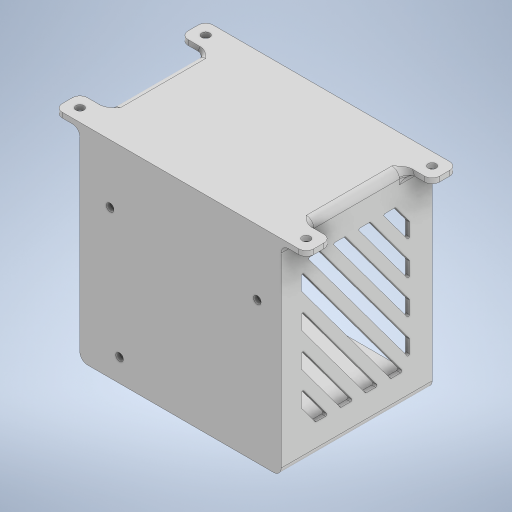
# Autodesk Inventor part: Caja2
Saved by Autodesk Inventor 2024 (Build 280153000, 153)
## iProperties
Created: 2023-04-03
Part Number: Caja2
Material: Genérico
Document SubType Name: Modeling
Designer: sergi
Density: 1 g/cm^3
Appearance: Valor por defecto
Author: sergi
Autodesk Inventor part; units mm, degrees
ref_plane "YZ Plane" through (0, 0, 0) normal (1, 0, 0) x (0, 1, 0)
ref_plane "XZ Plane" through (0, 0, 0) normal (0, 1, 0) x (-1, 0, 0)
ref_plane "XY Plane" through (0, 0, 0) normal (0, 0, 1) x (1, 0, 0)
sketch "Boceto1" plane through (0, 0, 0) normal (0, 0, 1) x (1, 0, 0)
  circle A0 centre (-35.8, -35.8) radius 2.125 projected
  circle A1 centre (35.8, 35.8) radius 2.125 projected
  circle A2 centre (35.8, -35.8) radius 2.125 projected
  circle A3 centre (-35.8, 35.8) radius 2.125 projected
  line L0 (-40, -40) -> (-40, 40) projected
  line L1 (40, -40) -> (-40, -40) projected
  line L2 (40, 40) -> (40, -40) projected
  line L3 (-40, 40) -> (40, 40) projected
  line L4 (-40, 40) -> (40, 40)
  line L5 (40, 40) -> (40, -40)
  line L6 (40, -40) -> (-40, -40)
  line L7 (-40, -40) -> (-40, 40)
  line L8 (-41, -41) -> (-41, 41)
  line L9 (-41, 41) -> (41, 41)
  line L10 (41, 41) -> (41, -41)
  line L11 (41, -41) -> (-41, -41)
  point P0 (0, 0)
  dimension "d22" = 1
  constraints: 16 end point, 2 parallel, 1 horizontal, 1 perpendicular, 3 other
  measures "d22" distance between parallel lines of L1 L11
extrude "Extrusión1" add sketch "Boceto1" along normal blind 60 contours A0 | A1 | A2 | A3 | L0 L3 L2 L1
sketch "Boceto2" plane through (0, 0, 0) normal (0, 0, -1) x (-1, 0, 0)
  circle A0 centre (35.8, 35.8) radius 2.125 projected
  circle A1 centre (35.8, -35.8) radius 2.125 projected
  circle A2 centre (-35.8, -35.8) radius 2.125 projected
  circle A3 centre (-35.8, 35.8) radius 2.125 projected
  point P0 (0, 0)
hole "Agujero1" at (-35.8, 35.8, 0) at (-35.8, -35.8, 0) at (35.8, -35.8, 0) at (35.8, 35.8, 0) direction (0, 0, 1) diameter 4.25 depth 10
shell "Vaciado1" thickness 1.6 removed faces 2 at (11.4636, -11.4031, 0) at (13.3333, 40, 20)
sketch "Boceto3" plane through (37.8, 37.8, 58.4) normal (0, 0, -1) x (-1, 0, 0)
  circle A0 centre (65.77, -19.059) radius 1.4999 projected
  circle A1 centre (62.025, -68.7162) radius 1.5 projected
  line L0 (76.2, 2.2) -> (76.2, -76.2) projected
  line L1 (-0.6, -76.2) -> (-0.6, 2.2) projected
  line L2 (76.2, -76.2) -> (-0.6, -76.2) projected
  circle A2 centre (7.8236, -54.3604) radius 1.5 projected
  circle A3 centre (7.2748, -21.6806) radius 1.5001 projected
  circle A4 centre (65.77, -19.059) radius 3
  circle A5 centre (62.025, -68.7162) radius 3
  circle A6 centre (7.8236, -54.3604) radius 3
  circle A7 centre (7.2748, -21.6806) radius 3
  line L3 (-0.6, 2.2) -> (76.2, 2.2) projected
  point P0 (37.8, -37.8)
  dimension "d10" = 6
  dimension "d11" = 6
  dimension "d12" = 6
  dimension "d13" = 6
  constraints: 4 centre point, 4 coincident
  measures "d10" diameter of A4
  measures "d11" diameter of A5
  measures "d12" diameter of A6
  measures "d13" diameter of A7
extrude "Extrusión2" add sketch "Boceto3" along normal blind 5 contours A4 | A5 | A6 | A7
fillet "Empalme1" radius 2 4 edges at (-21.225, -30.9162, 58.4) (32.9764, -16.5604, 58.4) (33.5252, 16.1194, 58.4) (-24.97, 18.741, 58.4)
sketch "Boceto4" plane through (-38.4, -38.4, 58.4) normal (1, 0, 0) x (0, 0, -1)
  line L0 (14.2955, 15.5019) -> (14.2955, 22.9876) projected
  line L1 (14.2955, 22.9876) -> (7, 23.1181) projected
  line L2 (7, 15.5019) -> (14.2955, 15.5019) projected
  line L3 (14.2955, 15.5019) -> (7, 15.5019)
  line L4 (7, 15.5019) -> (7, 23.1181)
  line L5 (7, 23.1181) -> (14.2955, 23.1181)
  line L6 (14.2955, 23.1181) -> (14.2955, 15.5019)
  line L7 (6, 24.1181) -> (6, 14.5019)
  line L8 (6, 14.5019) -> (15.2955, 14.5019)
  line L9 (15.2955, 14.5019) -> (15.2955, 24.1181)
  line L10 (15.2955, 24.1181) -> (6, 24.1181)
  point P0 (58.4, 38.4)
  point P1 (14.2955, 22.9876)
  point P2 (10.9796, 28.9019)
  dimension "d17" = 1
  constraints: 16 end point, 4 parallel, 2 perpendicular, 1 horizontal, 3 other
  measures "d17" distance between parallel lines of L4 L7
extrude "Extrusión3" cut sketch "Boceto4" against normal blind 5 contours L2 L4 L1 L0 | L1 L5 L6 | L10 L9 L8 L7
sketch "Boceto5" plane through (-40, 40, 0) normal (0, 1, 0) x (1, 0, 0)
  line L0 (0, -60) -> (80, -60) projected
  line L1 (0, -60) -> (80, -60)
  line L2 (80, -60) -> (80, 15.124)
  line L3 (80, 15.124) -> (0, 15.124)
  line L4 (0, 15.124) -> (0, -60)
  point P0 (40, 0)
  constraints: 8 end point, 2 parallel, 1 horizontal, 1 perpendicular
extrude "Extrusión4" add sketch "Boceto5" along normal blind 2
sketch "Boceto6" plane through (-40, 42, 0) normal (0, 1, 0) x (1, 0, 0)
  line L0 (80, 15.124) -> (0, 15.124) projected
  line L1 (80, -60) -> (80, 15.124) projected
  line L2 (0, 15.124) -> (80, 15.124)
  line L3 (80, 15.124) -> (80, 12.124)
  line L4 (80, 12.124) -> (0, 12.124)
  line L5 (0, 12.124) -> (0, 15.124)
  point P0 (40, 0)
  dimension "d25" = 3
  constraints: 8 end point, 2 parallel, 1 horizontal, 1 perpendicular, 1 point on line
  measures "d25" distance of L2.end L3.end
extrude "Extrusión5" add sketch "Boceto6" along normal blind 15
sketch "Boceto7" plane through (40, 40, -15.124) normal (0, 0, -1) x (-1, 0, 0)
  line L0 (0, 2) -> (80, 2) projected
  line L1 (80, 0) -> (80, 17) projected
  point P0 (40, -40)
  point P1 (70, 11.3)
  dimension "d28" = 9.3
  dimension "d29" = 10
  measures "d28" distance from line of L0 point (70, 11.3)
  measures "d29" distance from line of L1 point (70, 11.3)
hole "Agujero2" at (-30, 51.3, -15.124) direction (0, 0, 1) diameter 5 depth 10
sketch "Boceto8" plane through (40, 40, -15.124) normal (0, 0, -1) x (-1, 0, 0)
  line L0 (0, 2) -> (80, 2) projected
  line L1 (0, 0) -> (0, 17) projected
  point P0 (40, -40)
  point P1 (10, 11.3)
  dimension "d37" = 9.3
  dimension "d38" = 10
  measures "d37" distance from line of L0 point (10, 11.3)
  measures "d38" distance from line of L1 point (10, 11.3)
hole "Agujero3" at (30, 51.3, -15.124) direction (0, 0, 1) diameter 5 depth 10
fillet "Empalme2" radius 3 6 edges at (-40, 42, 23.938) (-40, -40, 30) (40, 42, 23.938) (40, -40, 30) (-40, 57, -13.624) (40, 57, -13.624)
sketch "Boceto9" plane through (-38.4, -33.1325, 0) normal (1, 0, 0) x (0, 0, -1)
  line L0 (-32.0511, 38.9222) -> (-32.0511, 48.6464) projected
  line L1 (-32.0511, 48.6464) -> (-43.4, 48.6464) projected
  line L2 (-58.4, 73.1325) -> (0, 73.1325) projected
  line L3 (-32.0511, 48.6464) -> (-7.565, 48.6464) construction
  line L4 (-42.05, 61.453) -> (-53.55, 61.453)
  line L5 (-53.55, 61.453) -> (-53.55, 70.953)
  line L6 (-53.55, 70.953) -> (-42.05, 70.953)
  line L7 (-42.05, 70.953) -> (-42.05, 61.453)
  line L8 (-58.4, 73.1325) -> (-58.4, -5.2675) projected
  point P0 (0, 33.1325)
  point P1 (-53.55, 66.203)
  dimension "d50" = 11.5
  dimension "d145" = 4.85
  dimension "d146" = 9.5
  constraints: 10 end point, 2 horizontal, 2 parallel, 1 midpoint, 1 perpendicular
  measures "d50" distance of L5.end L6.end
  measures "d145" distance between parallel lines of L8 L5
  measures "d146" distance of L6.end L4.start
extrude "Extrusión6" cut sketch "Boceto9" against normal blind 15
fillet "Empalme4" radius 2 6 edges at (33.1325, -38.4, 5.8) (38.4, -33.1325, 5.8) (38.4, 33.1325, 5.8) (-38.4, 33.1325, 5.8) (-33.1325, -38.4, 5.8) (-38.4, -33.1325, 5.8)
sketch "Boceto11" plane through (-38.4, -38.4, 58.4) normal (0, 1, 0) x (1, 0, 0)
  line L0 (17.175, 5) -> (11.175, 5) projected
  line L1 (17.175, 5) -> (67.175, 5)
  line L2 (67.175, 5) -> (67.175, 13)
  line L3 (67.175, 13) -> (17.175, 13)
  line L4 (17.175, 13) -> (17.175, 5)
  line L5 (71.3764, 5) -> (65.3764, 5) projected
  point P0 (38.4, 58.4)
  dimension "d58" = 50
  dimension "d59" = 8
  constraints: 8 end point, 2 parallel, 1 horizontal, 1 perpendicular
  measures "d58" distance of L3.end L2.end
  measures "d59" distance of L2.end L1.end
extrude "Extrusión8" cut sketch "Boceto11" against normal blind 4.5
ref_plane "Plano de trabajo1" through (0, 0, 0) normal (0, 0, -1) x (-1, 0, 0)
split "Dividir1" plane through (0, 0, 0) removes the side toward (0, 0, -1)
sketch "Boceto12" plane through (40, -37, 0) normal (1, 0, 0) x (0, 0, -1)
  line L0 (0, 0) -> (-60, 0) projected
  line L1 (0, 0) -> (0, 76) projected
  line L2 (-60, 76) -> (0, 76) projected
  line L3 (-60, 0) -> (-60, 76) projected
  line L4 (0, 106.0697) -> (0, -25.6754) projected
  line L5 (-51.3248, 9) -> (-9, 9)
  line L6 (-9, 9) -> (-9, 67)
  line L7 (-9, 67) -> (-50, 67)
  line L8 (-52, 0) -> (-52, 76)
  line L9 (-9, 9) -> (-52, 67)
  line L10 (-11.4897, 9) -> (-53.6066, 65.8089)
  line L11 (-9, 12.3582) -> (-50.3934, 68.1911)
  line L12 (-7.438, 16.9677) -> (-47.1801, 70.5734)
  line L13 (-4.2248, 19.3499) -> (-43.9669, 72.9556)
  line L14 (-1.0115, 21.7322) -> (-40.7536, 75.3378)
  line L15 (2.2017, 24.1144) -> (-37.5404, 77.7201)
  line L16 (5.415, 26.4967) -> (-34.3271, 80.1023)
  line L17 (8.6282, 28.8789) -> (-31.1139, 82.4845)
  line L18 (-16.4691, 9) -> (-56.8199, 63.4266)
  line L19 (-20.291, 7.4388) -> (-60.0331, 61.0444)
  line L20 (-23.5043, 5.0565) -> (-63.2464, 58.6622)
  line L21 (-26.7175, 2.6743) -> (-66.4596, 56.2799)
  line L22 (-29.9307, 0.2921) -> (-69.6729, 53.8977)
  line L23 (-33.144, -2.0902) -> (-72.8861, 51.5155)
  line L24 (-36.3572, -4.4724) -> (-76.0994, 49.1332)
  line L25 (11.8415, 31.2611) -> (-27.9006, 84.8668)
  line L26 (15.0547, 33.6434) -> (-24.6874, 87.249)
  line L27 (-39.5705, -6.8546) -> (-79.3126, 46.751)
  point P0 (-42, 9)
  point P1 (-41.366, 9)
  point P2 (-52, 23.3435)
  point P3 (-9, 19.0746)
  point P4 (-44.5309, 67)
  point P5 (-49.5103, 67)
  point P6 (-9, 13.0443)
  point P7 (-9, 32.5073)
  point P8 (-34.5721, 67)
  point P9 (-39.5515, 67)
  point P10 (-9, 25.791)
  point P11 (-9, 45.9401)
  point P12 (-24.6134, 67)
  point P13 (-29.5928, 67)
  point P14 (-9, 39.2237)
  point P15 (-19.634, 67)
  point P16 (-9, 52.6565)
  point P17 (-52, 56.9254)
  point P18 (-15.9032, 9)
  point P19 (-11.3011, 9)
  point P20 (-52, 63.6418)
  point P21 (-52, 43.4927)
  point P22 (-26.4279, 9)
  point P23 (-21.4485, 9)
  point P24 (-52, 50.209)
  point P25 (-52, 30.0599)
  point P26 (-36.3866, 9)
  point P27 (-31.4072, 9)
  point P28 (-52, 36.7763)
  point P29 (-52, 16.6271)
  point P30 (-46.3454, 9)
  point P31 (-9, 59.3729)
  point P32 (-14.6546, 67)
  dimension "d83" = 9
  dimension "d84" = 8
  dimension "L" = 2
  dimension "d86" = 2
  dimension "d87" = 4
  dimension "d88" = 4
  dimension "d89" = 4
  dimension "d90" = 4
  dimension "d91" = 4
  dimension "d92" = 4
  dimension "d93" = 4
  dimension "d94" = 4
  dimension "d95" = 4
  dimension "d96" = 4
  dimension "d97" = 4
  dimension "d98" = 4
  dimension "d99" = 4
  dimension "d140" = 4
  dimension "d141" = 4
  dimension "d142" = 4
  constraints: 46 end point, 19 parallel, 6 point on line, 1 other
  measures "d83" distance between parallel lines of L0 L5
  measures "d84" distance between parallel lines of L3 L8
  measures "L" distance between parallel lines of L9 L10
  measures "d86" distance between parallel lines of L9 L11
  measures "d87" distance between parallel lines of L11 L12
  measures "d88" distance between parallel lines of L12 L13
  measures "d89" distance between parallel lines of L13 L14
  measures "d90" distance between parallel lines of L14 L15
  measures "d91" distance between parallel lines of L15 L16
  measures "d92" distance between parallel lines of L16 L17
  measures "d93" distance between parallel lines of L10 L18
  measures "d94" distance between parallel lines of L18 L19
  measures "d95" distance between parallel lines of L19 L20
  measures "d96" distance between parallel lines of L20 L21
  measures "d97" distance between parallel lines of L21 L22
  measures "d98" distance between parallel lines of L22 L23
  measures "d99" distance between parallel lines of L23 L24
  measures "d140" distance between parallel lines of L17 L25
  measures "d141" distance between parallel lines of L25 L26
  measures "d142" distance between parallel lines of L24 L27
extrude "Extrusión9" cut sketch "Boceto12" against normal up to surface (1.6 mm away) contours L8 L23 L5 L24 | L8 L21 L5 L22 | L15 L7 L16 L6 | L8 L19 L5 L20 | L6 L13 L7 L14 | L17 L7 L25 L6 | L8 L10 L5 L18 | L6 L11 L7 L12
fillet "Empalme5" radius 0.5 32 edges at (39.2, -17.9254, 9) (39.2, -28, 21.4485) (39.2, -28, 26.4279) (39.2, -28, 31.4072) (39.2, -28, 36.3866) (39.2, -28, 41.366) (39.2, -13.6565, 52) (39.2, -6.9401, 52) (39.2, -0.2237, 52) (39.2, 6.4927, 52) (39.2, 13.209, 52) (39.2, 19.9254, 52) (39.2, 26.6418, 52) (39.2, 30, 49.5103) (39.2, 30, 44.5309) (39.2, 30, 39.5515) (39.2, 30, 34.5721) (39.2, 30, 29.5928) (39.2, 30, 24.6134) (39.2, 30, 19.634) (39.2, 15.6565, 9) (39.2, 8.9401, 9) (39.2, 2.2237, 9) (39.2, -4.4927, 9) (39.2, -11.209, 9) (39.2, -24.6418, 9) (39.2, -28, 11.4897) (39.2, -28, 16.4691) (39.2, -28, 46.3454) (39.2, -20.3729, 52) (39.2, 30, 14.6546) (39.2, 22.3729, 9)
sketch "Boceto13" plane through (-40, -37, 0) normal (-1, 0, 0) x (0, 0, 1)
  line L0 (36.5365, 9.2022) -> (51.9017, 29.9272) construction
  arc A0 (51.9017, 29.9272) -> (52, 30.225) centre (51.5, 30.225) ccw construction
  line L1 (52, 30.225) -> (52, 35.2623) construction
  arc A1 (52, 35.2623) -> (51.0983, 35.5601) centre (51.5, 35.2623) ccw construction
  line L2 (51.0983, 35.5601) -> (31.9987, 9.7978) construction
  arc A2 (31.9987, 9.7978) -> (32.4004, 9) centre (32.4004, 9.5) ccw construction
  line L3 (32.4004, 9) -> (36.1349, 9) construction
  arc A3 (36.1349, 9) -> (36.5365, 9.2022) centre (36.1349, 9.5) ccw construction
  line L4 (28.5996, 67) -> (24.8651, 67) construction
  line L5 (9, 45.775) -> (9, 40.7377) construction
  line L6 (26.5778, 9.2022) -> (51.9017, 43.36) construction
  arc A4 (51.9017, 43.36) -> (52, 43.6578) centre (51.5, 43.6578) ccw construction
  line L7 (52, 43.6578) -> (52, 48.6951) construction
  arc A5 (52, 48.6951) -> (51.0983, 48.9929) centre (51.5, 48.6951) ccw construction
  line L8 (51.0983, 48.9929) -> (22.0399, 9.7978) construction
  arc A6 (22.0399, 9.7978) -> (22.4416, 9) centre (22.4416, 9.5) ccw construction
  line L9 (22.4416, 9) -> (26.1761, 9) construction
  arc A7 (26.1761, 9) -> (26.5778, 9.2022) centre (26.1761, 9.5) ccw construction
  line L10 (44.381, 66.7978) -> (9.0983, 19.2072) construction
  arc A8 (9.0983, 19.2072) -> (9, 18.9094) centre (9.5, 18.9094) ccw construction
  arc A9 (44.7827, 67) -> (44.381, 66.7978) centre (44.7827, 66.5) ccw construction
  line L11 (0, 0) -> (60, 0) construction
  line L12 (0, 0) -> (0, 76) construction
  line L13 (60, 76) -> (0, 76) construction
  line L14 (60, 0) -> (60, 76) construction
  line L15 (24.4635, 66.7978) -> (9.0983, 46.0728) construction
  arc A10 (9.0983, 46.0728) -> (9, 45.775) centre (9.5, 45.775) ccw construction
  arc A11 (9, 40.7377) -> (9.9017, 40.4399) centre (9.5, 40.7377) ccw construction
  line L16 (9.9017, 40.4399) -> (29.0013, 66.2022) construction
  arc A12 (29.0013, 66.2022) -> (28.5996, 67) centre (28.5996, 66.5) ccw construction
  arc A13 (24.8651, 67) -> (24.4635, 66.7978) centre (24.8651, 66.5) ccw construction
  line L17 (48.5172, 67) -> (44.7827, 67) construction
  line L18 (9, 59.2077) -> (9, 54.1705) construction
  line L19 (9.9017, 13.5744) -> (48.9188, 66.2022) construction
  arc A14 (48.9188, 66.2022) -> (48.5172, 67) centre (48.5172, 66.5) ccw construction
  line L20 (14.5047, 66.7978) -> (9.0983, 59.5055) construction
  arc A15 (9.0983, 59.5055) -> (9, 59.2077) centre (9.5, 59.2077) ccw construction
  arc A16 (9, 54.1705) -> (9.9017, 53.8727) centre (9.5, 54.1705) ccw construction
  line L21 (9.9017, 53.8727) -> (19.0425, 66.2022) construction
  arc A17 (19.0425, 66.2022) -> (18.6409, 67) centre (18.6409, 66.5) ccw construction
  line L22 (18.6409, 67) -> (14.9063, 67) construction
  arc A18 (14.9063, 67) -> (14.5047, 66.7978) centre (14.9063, 66.5) ccw construction
  line L23 (38.5584, 67) -> (34.8239, 67) construction
  arc A19 (34.8239, 67) -> (34.4222, 66.7978) centre (34.8239, 66.5) ccw construction
  line L24 (34.4222, 66.7978) -> (9.0983, 32.64) construction
  arc A20 (9.0983, 32.64) -> (9, 32.3422) centre (9.5, 32.3422) ccw construction
  line L25 (9, 32.3422) -> (9, 27.3049) construction
  arc A21 (9, 27.3049) -> (9.9017, 27.0071) centre (9.5, 27.3049) ccw construction
  line L26 (9.9017, 27.0071) -> (38.9601, 66.2022) construction
  arc A22 (38.9601, 66.2022) -> (38.5584, 67) centre (38.5584, 66.5) ccw construction
  line L27 (9, 18.9094) -> (9, 13.8722) construction
  arc A23 (9, 13.8722) -> (9.9017, 13.5744) centre (9.5, 13.8722) ccw construction
  line L28 (12.4828, 9) -> (16.2173, 9) projected
  arc A24 (16.2173, 9) -> (16.619, 9.2022) centre (16.2173, 9.5) ccw projected
  line L29 (16.619, 9.2022) -> (51.9017, 56.7928) projected
  arc A25 (51.9017, 56.7928) -> (52, 57.0906) centre (51.5, 57.0906) ccw projected
  line L30 (52, 57.0906) -> (52, 62.1278) projected
  arc A26 (52, 62.1278) -> (51.0983, 62.4256) centre (51.5, 62.1278) ccw projected
  line L31 (51.0983, 62.4256) -> (12.0812, 9.7978) projected
  arc A27 (12.0812, 9.7978) -> (12.4828, 9) centre (12.4828, 9.5) ccw projected
  line L32 (14.5047, 66.7978) -> (9.0983, 59.5055) projected
  arc A28 (9.0983, 59.5055) -> (9, 59.2077) centre (9.5, 59.2077) ccw projected
  line L33 (9, 59.2077) -> (9, 54.1705) projected
  arc A29 (9, 54.1705) -> (9.9017, 53.8727) centre (9.5, 54.1705) ccw projected
  line L34 (9.9017, 53.8727) -> (19.0425, 66.2022) projected
  arc A30 (19.0425, 66.2022) -> (18.6409, 67) centre (18.6409, 66.5) ccw projected
  line L35 (18.6409, 67) -> (14.9063, 67) projected
  arc A31 (14.9063, 67) -> (14.5047, 66.7978) centre (14.9063, 66.5) ccw projected
  line L36 (38.5584, 67) -> (34.8239, 67) projected
  arc A32 (34.8239, 67) -> (34.4222, 66.7978) centre (34.8239, 66.5) ccw projected
  line L37 (34.4222, 66.7978) -> (9.0983, 32.64) projected
  arc A33 (9.0983, 32.64) -> (9, 32.3422) centre (9.5, 32.3422) ccw projected
  line L38 (9, 32.3422) -> (9, 27.3049) projected
  arc A34 (9, 27.3049) -> (9.9017, 27.0071) centre (9.5, 27.3049) ccw projected
  line L39 (9.9017, 27.0071) -> (38.9601, 66.2022) projected
  arc A35 (38.9601, 66.2022) -> (38.5584, 67) centre (38.5584, 66.5) ccw projected
  line L40 (26.5778, 9.2022) -> (51.9017, 43.36) projected
  arc A36 (51.9017, 43.36) -> (52, 43.6578) centre (51.5, 43.6578) ccw projected
  line L41 (52, 43.6578) -> (52, 48.6951) projected
  arc A37 (52, 48.6951) -> (51.0983, 48.9929) centre (51.5, 48.6951) ccw projected
  line L42 (51.0983, 48.9929) -> (22.0399, 9.7978) projected
  arc A38 (22.0399, 9.7978) -> (22.4416, 9) centre (22.4416, 9.5) ccw projected
  line L43 (22.4416, 9) -> (26.1761, 9) projected
  arc A39 (26.1761, 9) -> (26.5778, 9.2022) centre (26.1761, 9.5) ccw projected
  line L44 (48.5172, 67) -> (44.7827, 67) projected
  arc A40 (44.7827, 67) -> (44.381, 66.7978) centre (44.7827, 66.5) ccw projected
  line L45 (44.381, 66.7978) -> (9.0983, 19.2072) projected
  arc A41 (9.0983, 19.2072) -> (9, 18.9094) centre (9.5, 18.9094) ccw projected
  line L46 (9, 18.9094) -> (9, 13.8722) projected
  arc A42 (9, 13.8722) -> (9.9017, 13.5744) centre (9.5, 13.8722) ccw projected
  line L47 (9.9017, 13.5744) -> (48.9188, 66.2022) projected
  arc A43 (48.9188, 66.2022) -> (48.5172, 67) centre (48.5172, 66.5) ccw projected
  line L48 (46.4953, 9.2022) -> (51.9017, 16.4945) projected
  arc A44 (51.9017, 16.4945) -> (52, 16.7923) centre (51.5, 16.7923) ccw projected
  line L49 (52, 16.7923) -> (52, 21.8295) projected
  arc A45 (52, 21.8295) -> (51.0983, 22.1273) centre (51.5, 21.8295) ccw projected
  line L50 (51.0983, 22.1273) -> (41.9575, 9.7978) projected
  arc A46 (41.9575, 9.7978) -> (42.3591, 9) centre (42.3591, 9.5) ccw projected
  line L51 (42.3591, 9) -> (46.0937, 9) projected
  arc A47 (46.0937, 9) -> (46.4953, 9.2022) centre (46.0937, 9.5) ccw projected
  line L52 (28.5996, 67) -> (24.8651, 67) projected
  arc A48 (24.8651, 67) -> (24.4635, 66.7978) centre (24.8651, 66.5) ccw projected
  line L53 (24.4635, 66.7978) -> (9.0983, 46.0728) projected
  arc A49 (9.0983, 46.0728) -> (9, 45.775) centre (9.5, 45.775) ccw projected
  line L54 (9, 45.775) -> (9, 40.7377) projected
  arc A50 (9, 40.7377) -> (9.9017, 40.4399) centre (9.5, 40.7377) ccw projected
  line L55 (9.9017, 40.4399) -> (29.0013, 66.2022) projected
  arc A51 (29.0013, 66.2022) -> (28.5996, 67) centre (28.5996, 66.5) ccw projected
  line L56 (36.5365, 9.2022) -> (51.9017, 29.9272) projected
  arc A52 (51.9017, 29.9272) -> (52, 30.225) centre (51.5, 30.225) ccw projected
  line L57 (52, 30.225) -> (52, 35.2623) projected
  arc A53 (52, 35.2623) -> (51.0983, 35.5601) centre (51.5, 35.2623) ccw projected
  line L58 (51.0983, 35.5601) -> (31.9987, 9.7978) projected
  arc A54 (31.9987, 9.7978) -> (32.4004, 9) centre (32.4004, 9.5) ccw projected
  line L59 (32.4004, 9) -> (36.1349, 9) projected
  arc A55 (36.1349, 9) -> (36.5365, 9.2022) centre (36.1349, 9.5) ccw projected
  line L60 (0, 0) -> (60, 0) projected
  line L61 (0, 0) -> (0, 76) projected
  line L62 (60, 76) -> (0, 76) projected
  line L63 (60, 0) -> (60, 76) projected
  line L64 (43.1045, 13.1019) -> (43.1045, 22.7181) projected
  line L65 (36.1045, 9) -> (36.1045, 67)
  point P0 (36.1045, 62.3505)
  point P1 (36.1045, 48.9177)
  point P2 (36.1045, 55.6341)
  point P3 (36.1045, 35.485)
  point P4 (36.1045, 42.2014)
  point P5 (36.1045, 22.0522)
  point P6 (36.1045, 28.7686)
  point P7 (36.1045, 15.3358)
  dimension "d143" = 7
  constraints: 2 end point, 2 point on line, 1 parallel
  measures "d143" distance between parallel lines of L64 L65
extrude "Extrusión10" cut sketch "Boceto13" against normal up to surface (1.6 mm away) contours A27 L31 L65 L29 A24 L28 | A31 L35 A30 L34 A29 L33 A28 L32 | L65 L39 A34 L38 A33 L37 A32 L36 | A39 L43 A38 L42 L65 L40 | L47 A42 L46 A41 L45 L65 | A51 L55 A50 L54 A49 L53 A48 L52 | L59 A54 L58 L65
sketch "Boceto14" plane through (-40, 42, 0) normal (0, 1, 0) x (1, 0, 0)
  line L0 (77, 0) -> (3, 0) projected
  line L1 (3, -60) -> (3, 0) projected
  line L2 (3, -60) -> (77, -60) projected
  line L3 (77, 0) -> (77, -60) projected
  line L4 (0, 0) -> (0, -60) projected
  line L5 (80, -60) -> (80, 0) projected
  line L6 (80, -60) -> (77, -60) projected
  line L7 (-30, 0) -> (110, 0) projected
  line L8 (3, -60) -> (0, -60) projected
  line L9 (0, 0) -> (-10, 0)
  line L10 (-10, 0) -> (-10, -10)
  line L11 (-10, -10) -> (0, -10)
  line L12 (0, -10) -> (0, 0)
  line L13 (0, -60) -> (-10, -60)
  line L14 (-10, -60) -> (-10, -50)
  line L15 (-10, -50) -> (0, -50)
  line L16 (0, -50) -> (0, -60)
  line L17 (0, -50) -> (3, -50)
  line L18 (0, -10) -> (3, -10)
  line L19 (80, -60) -> (90, -60)
  line L20 (90, -60) -> (90, -50)
  line L21 (90, -50) -> (80, -50)
  line L22 (80, -50) -> (80, -60)
  line L23 (80, 0) -> (90, 0)
  line L24 (90, 0) -> (90, -10)
  line L25 (90, -10) -> (80, -10)
  line L26 (80, -10) -> (80, 0)
  line L27 (80, -10) -> (77, -10)
  line L28 (80, -50) -> (77, -50)
  point P0 (40, 0)
  dimension "d105" = 10
  dimension "d106" = 10
  dimension "d107" = 10
  dimension "d108" = 10
  dimension "d109" = 10
  dimension "d110" = 10
  dimension "d111" = 10
  dimension "d112" = 10
  constraints: 40 end point, 9 parallel, 7 perpendicular, 4 horizontal, 4 point on line
  measures "d105" distance of L11.end L10.end
  measures "d106" distance of L10.end L9.end
  measures "d107" distance of L14.end L15.end
  measures "d108" distance of L13.end L14.end
  measures "d109" distance of L21.end L20.end
  measures "d110" distance of L20.end L19.end
  measures "d111" distance of L24.end L25.end
  measures "d112" distance of L23.end L24.end
extrude "Extrusión11" add sketch "Boceto14" against normal blind 2 contours L7 L5 L27 L3 | L1 L18 L4 L7 | L7 L24 L25 L5 | L4 L11 L10 L7 | L28 L5 L6 L3 | L1 L8 L4 L17 | L21 L20 L19 L5 | L4 L13 L14 L15
fillet "Empalme7" radius 3 8 edges at (-50, 41, 0) (-50, 41, 10) (-50, 41, 50) (-50, 41, 60) (50, 41, 0) (50, 41, 10) (50, 41, 50) (50, 41, 60)
fillet "Empalme8" radius 3 4 edges at (-39.8284, 40, 55) (-39.8284, 40, 5) (39.8284, 40, 5) (39.8284, 40, 55)
sketch "Boceto15" plane through (-40, 40, 0) normal (0, -1, 0) x (1, 0, 0)
  line L0 (90, 3) -> (90, 7) projected
  line L1 (83, 0) -> (87, 0) projected
  line L2 (90, 53) -> (90, 57) projected
  line L3 (83, 50) -> (87, 50) projected
  line L4 (-10, 7) -> (-10, 3) projected
  line L5 (-7, 0) -> (-3, 0) projected
  line L6 (-10, 57) -> (-10, 53) projected
  line L7 (-3, 60) -> (-7, 60) projected
  point P0 (40, 0)
  point P1 (85, 5)
  point P2 (85, 55)
  point P3 (-5, 5)
  point P4 (-5, 55)
  dimension "d117" = 5
  dimension "d118" = 5
  dimension "d119" = 5
  dimension "d120" = 5
  dimension "d121" = 5
  dimension "d122" = 5
  dimension "d123" = 5
  dimension "d124" = 5
  measures "d117" distance from line of L0 point (85, 5)
  measures "d118" distance from line of L1 point (85, 5)
  measures "d119" distance from line of L2 point (85, 55)
  measures "d120" distance from line of L3 point (85, 55)
  measures "d121" distance from line of L4 point (-5, 5)
  measures "d122" distance from line of L5 point (-5, 5)
  measures "d123" distance from line of L6 point (-5, 55)
  measures "d124" distance from line of L7 point (-5, 55)
hole "Agujero4" at (45, 40, 5) at (45, 40, 55) at (-45, 40, 5) at (-45, 40, 55) direction (0, 1, 0) diameter 3.2 end through all
sketch "Boceto16" plane through (-27.97, 18.741, 58.4) normal (0, 0, -1) x (-1, 0, 0)
  circle A0 centre (0, 0) radius 1.4999 projected
  circle A1 centre (-58.4952, -2.6215) radius 1.5001 projected
  circle A2 centre (-3.745, -49.6572) radius 1.5 projected
  point P0 (-27.97, -18.741)
  constraints: 3 coincident
hole "Agujero5" at (-27.97, 18.741, 58.4) at (30.5252, 16.1194, 58.4) at (-24.225, -30.9162, 58.4) direction (0, 0, 1) diameter 3 end through all
fillet "Empalme9" radius 3 8 edges at (-40, 38.4103, 50) (-39.1213, 41.1213, 50) (-40, 38, 10) (-39.1213, 41.1213, 10) (40, 38, 50) (39.1213, 41.1213, 50) (40, 38, 10) (39.1213, 41.1213, 10)
fillet "Empalme10" radius 0.5 10 edges at (-39.2, -21.6642, 36.1045) (-39.2, -28, 36.1045) (-39.2, -14.9478, 36.1045) (-39.2, -8.2314, 36.1045) (-39.2, -1.515, 36.1045) (-39.2, 5.2014, 36.1045) (-39.2, 18.6341, 36.1045) (-39.2, 11.9177, 36.1045) (-39.2, 25.3505, 36.1045) (-39.2, 30, 36.1045)
sketch "Boceto17" plane through (38.4, -38.4, 58.4) normal (0, 0, -1) x (-1, 0, 0)
  line L0 (76.8, 66.7206) -> (76.8, 76.2206) projected
  line L1 (76.8, 66.7206) -> (61.8, 66.7206)
  line L2 (61.8, 66.7206) -> (61.8, 76.2206)
  line L3 (61.8, 76.2206) -> (76.8, 76.2206)
  line L4 (76.8, 76.2206) -> (76.8, 66.7206)
  point P0 (38.4, 38.4)
  dimension "d148" = 15
  constraints: 8 end point, 2 parallel, 1 horizontal, 1 perpendicular
  measures "d148" distance of L2.end L3.end
extrude "Extrusión12" add sketch "Boceto17" along normal up to surface (4.85 mm away)
fillet "Empalme11" radius 1.5 4 edges at (28.775, -39.2, 53.4) (28.775, -39.2, 45.4) (-21.225, -39.2, 45.4) (-21.225, -39.2, 53.4)
equation "\"d86\" = L"
equation "\"d87\" = 2 * L"
equation "\"d88\" = 2 * L"
equation "\"d89\" = 2 * L"
equation "\"d90\" = 2 * L"
equation "\"d92\" = 2 * L"
equation "\"d93\" = 2 * L"
equation "\"d94\" = 2 * L"
equation "\"d95\" = 2 * L"
equation "\"d96\" = 2 * L"
equation "\"d97\" = 2 * L"
equation "\"d98\" = 2 * L"
equation "\"d99\" = 2 * L"
